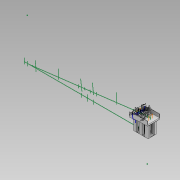
# Autodesk Inventor part: Slope_HighEnd
Saved by Autodesk Inventor 2021 (Build 250183000, 183)
## iProperties
Created: 2021-03-11
Part Number: Slope_HighEnd
Material: 一般
Document SubType Name: Modeling
Designer: kumagai
Density: 1 g/cm^3
Appearance: 既定
Author: kumagai
Autodesk Inventor part; units mm, degrees
ref_plane "YZ Plane" through (0, 0, 0) normal (1, 0, 0) x (0, 1, 0)
ref_plane "XZ Plane" through (0, 0, 0) normal (0, 1, 0) x (-1, 0, 0)
ref_plane "XY Plane" through (0, 0, 0) normal (0, 0, 1) x (1, 0, 0)
derived "SlopeProfile.ipt"
sketch "スケッチ1" plane through (0, 0, 0) normal (0, 0, 1) x (1, 0, 0)
  line L0 (0, 14) -> (0, -14)
  line L1 (-14, 0) -> (14, 0)
  line L2 (-268.75, 0) -> (268.75, 0)
  line L3 (-268.75, 0) -> (268.75, 66)
  line L4 (268.75, 66) -> (268.75, 0)
  line L5 (-31.5879, 61.457) -> (-25.6465, 13.0705)
  line L6 (-134.375, 50.6657) -> (-134.375, 8.5939)
  line L7 (23.2129, 72.7486) -> (28.7067, 28.0077)
  line L8 (-244.2356, 29.1492) -> (-240.1953, -3.7549)
  line L9 (134.375, 89.7324) -> (134.375, 45.3233)
  line L10 (239.1121, 78.5758) -> (241.9591, 55.3901)
  line L11 (-27.6764, 5.7379) -> (-27.6764, -11.9933)
  line L12 (27.6764, 6.5088) -> (27.6764, -13.0212)
  line L13 (-268.75, 0) -> (-295.625, 0)
  line L14 (268.75, 66) -> (295.625, 66)
  line L15 (241.0736, 6.6999) -> (241.0736, -9.2827)
  line L16 (-241.0736, -7.7427) -> (-241.0736, -14.414)
  arc A0 (-280.625, 0) -> (-256.9635, 1.4473) centre (-280.625, 194.1449) ccw
  line L17 (-256.3082, 4.3915) -> (-255.7778, 0.0713)
  line L18 (-280.625, 8.6126) -> (-280.625, -11.6883)
  line L19 (-295.625, 14.7784) -> (-295.625, -11.568)
  line L20 (255.3892, 69.0933) -> (256.9398, 56.465)
  line L21 (280.625, 71.1514) -> (280.625, 58.4982)
  line L22 (295.625, 71.9522) -> (295.625, 60.0478)
  arc A1 (280.625, 66) -> (256.9635, 64.5527) centre (280.625, -128.1449) ccw
  line L23 (-13.2739, 35.3851) -> (-12.039, 25.3288)
  line L24 (-43.1495, 32.5373) -> (-41.4451, 18.6566)
  line L25 (12.2235, 39.1691) -> (13.7539, 26.7059)
  line L26 (41.8424, 44.108) -> (43.6336, 29.5201)
  point P0 (0, 0)
  point P1 (-241.0736, 3.3984)
  point P2 (-27.6764, 29.6016)
  point P3 (27.6764, 36.3984)
  point P4 (241.0736, 62.6016)
  point P5 (134.375, 49.5)
  point P6 (-134.375, 16.5)
ref_plane "作業平面1" through (241.0736, 62.6016, 0) normal (0.9925454, 0.1218753, 0) x (-0.1218753, 0.9925454, 0)
sketch "スケッチ2" plane through (241.0736, 62.6016, 0) normal (0.9925454, 0.1218753, 0) x (-0.1218753, 0.9925454, 0)
  line L0 (16.0942, 0) -> (-7.2657, 0) projected
  line L1 (3.2, 19) -> (-5.2, 19)
  line L2 (-5.2, 19) -> (-5.2, -19)
  line L3 (-5.2, -19) -> (3.2, -19)
  line L4 (3.2, -19) -> (3.2, -17)
  line L5 (3.2, -17) -> (0, -17)
  line L6 (0, -17) -> (0, -9.3)
  line L7 (0, -9.3) -> (3.2, -9.3)
  line L8 (3.2, -9.3) -> (3.2, -6.9)
  line L9 (3.2, -6.9) -> (0, -6.9)
  line L10 (0, -6.9) -> (0, 6.9)
  line L11 (0, 6.9) -> (3.2, 6.9)
  line L12 (3.2, 6.9) -> (3.2, 9.3)
  line L13 (3.2, 9.3) -> (0, 9.3)
  line L14 (0, 9.3) -> (0, 17)
  line L15 (0, 17) -> (3.2, 17)
  line L16 (3.2, 17) -> (3.2, 19)
  line L17 (-5.2, 27.5) -> (-5.2, -27.5)
  line L18 (-5.2, -27.5) -> (9, -27.5)
  line L19 (9, -27.5) -> (9, -29.5)
  line L20 (9, -29.5) -> (-11, -29.5)
  line L21 (-11, -29.5) -> (-11, 29.5)
  line L22 (-11, 29.5) -> (9, 29.5)
  line L23 (9, 29.5) -> (9, 27.5)
  line L24 (9, 27.5) -> (-5.2, 27.5)
  line L25 (-11, -29.5) -> (-20.0203, -18.75)
  line L26 (-20.0203, -18.75) -> (-31, -18.75)
  line L27 (-31, -18.75) -> (-31, -10.75)
  line L28 (-31, -10.75) -> (-20.0203, -10.75)
  line L29 (-20.0203, -10.75) -> (-11, 0)
  line L30 (-11, 0) -> (-20.0203, 10.75)
  line L31 (-20.0203, 10.75) -> (-31, 10.75)
  line L32 (-31, 10.75) -> (-31, 18.75)
  line L33 (-31, 18.75) -> (-20.0203, 18.75)
  line L34 (-20.0203, 18.75) -> (-11, 29.5)
  point P0 (-32.754, 0)
  point P1 (0, 0)
  point P2 (-5.2, 19)
  point P3 (-5.2, -19)
  dimension "d14" = 27.6764
  dimension "d25" = 38
  dimension "d26" = 8.4
  dimension "d27" = 3.2
  dimension "d28" = 18.6
  dimension "d29" = 2.4
  dimension "d30" = 2
  dimension "d31" = 59
  dimension "d32" = 2
  dimension "d33" = 20
  dimension "d34" = 5.8
  dimension "d36" = 5.8
  dimension "d53" = 40
  dimension "d54" = 40
  dimension "d55" = 8
  dimension "d56" = 20
  constraints: 68 end point, 21 perpendicular, 6 point on line, 3 collinear, 3 horizontal, 3 vertical, 2 midpoint, 1 parallel, 1 vertical alignment, 11 other
  measures "d25" distance between parallel lines of L3 L1
  measures "d26" distance between parallel lines of L2 L4
  measures "d27" distance between parallel lines of L6 L4
  measures "d28" distance between parallel lines of L7 L13
  measures "d29" distance between parallel lines of L13 L11
  measures "d30" distance between parallel lines of L1 L15
  measures "d31" distance between parallel lines of L22 L20
  measures "d32" distance between parallel lines of L22 L24
  measures "d33" distance between parallel lines of L21 L19
  measures "d34" distance between parallel lines of L4 L19
  measures "d36" distance between parallel lines of L21 L17
  measures "d53" angle of L21 L25
  measures "d54" angle of L21 L29
  measures "d55" distance between parallel lines of L28 L26
  measures "d56" distance between parallel lines of L27 L21
sketch "スケッチ3" plane through (0, 0, 0) normal (0, 0, 1) x (1, 0, 0)
  arc A0 (280.625, 66) -> (256.9635, 64.5527) centre (280.625, -128.1449) ccw projected
  line L0 (-268.75, 0) -> (268.75, 66) projected
  line L1 (256.9635, 64.5527) -> (226.1855, 60.7735)
  line L2 (239.1121, 78.5758) -> (241.9591, 55.3901) projected
  line L3 (280.625, 66) -> (310.625, 66)
  line L4 (295.625, 71.9522) -> (295.625, 60.0478) projected
  point P0 (0, 0)
  dimension "d14" = 27.6764
  dimension "d37" = 15
  dimension "d39" = 15
  constraints: 4 end point, 1 horizontal, 1 point on line
  measures "d37" distance from line of L1.end L2
  measures "d39" distance from line of L3.end L4
sweep "スイープ1" add profiles "スケッチ2" path "スケッチ3" path curves L1 A0 L3
extrude "押し出し1" cut sketch "スケッチ2" along normal blind 15 and the other way blind 15 contours L10 L9 L8 L7 L6 L5 L4 L3 L2 L0 | L0 L2 L1 L16 L15 L14 L13 L12 L11 L10
ref_plane "作業平面2" through (295.625, 66, 0) normal (1, 0, 0) x (0, 1, 0)
sketch "スケッチ4" plane through (295.625, 66, 0) normal (1, 0, 0) x (0, 1, 0)
  line L0 (3.2, 19.5) -> (-5.2, 19.5)
  line L1 (-5.2, 19.5) -> (-5.2, -19.5)
  line L2 (-5.2, -19.5) -> (3.2, -19.5)
  line L3 (3.2, -19.5) -> (3.2, 19.5)
  line L4 (5.9522, 0) -> (-5.9522, 0) projected
  point P0 (-66, 0)
  point P1 (0, 0)
  dimension "d14" = 27.6764
  dimension "d46" = 39
  dimension "d47" = 3.2
  dimension "d48" = 8.4
  constraints: 8 end point, 2 parallel, 1 horizontal, 1 perpendicular, 1 other
  measures "d46" distance between parallel lines of L2 L0
  measures "d47" distance from line of point (0, 0) L3
  measures "d48" distance between parallel lines of L1 L3
extrude "押し出し2" cut sketch "スケッチ4" along normal blind 15 and the other way blind 15
sketch "スケッチ5" plane through (295.625, 66, 0) normal (1, 0, 0) x (0, 1, 0)
  line L0 (-66, 41.3) -> (-66, -41.3) projected
  line L1 (-20.0203, 18.75) -> (-71.2, 18.75)
  line L2 (-71.2, 18.75) -> (-71.2, 10.75)
  line L3 (-69.2, 10.75) -> (-20.0203, 10.75)
  line L4 (-20.0203, 10.75) -> (-20.0203, 18.75)
  line L5 (-21.3183, -18.75) -> (-20.0203, -18.75) projected
  line L6 (-20.0203, -18.75) -> (-71.2, -18.75)
  line L7 (-71.2, -18.75) -> (-71.2, -10.75)
  line L8 (-69.2, -10.75) -> (-20.0203, -10.75)
  line L9 (-20.0203, -10.75) -> (-20.0203, -18.75)
  line L10 (-258.6029, 0) -> (192.6029, 0) projected
  line L11 (-71.2, -10.75) -> (-71.2, 10.75)
  line L12 (-69.2, -10.75) -> (-69.2, 10.75)
  point P0 (-66, 0)
  dimension "d57" = 5.2
  dimension "d76" = 2
  constraints: 20 end point, 5 parallel, 2 horizontal, 2 perpendicular, 2 point on line, 1 vertical, 2 other
  measures "d57" distance between parallel lines of L0 L2
  measures "d76" distance between parallel lines of L11 L12
extrude "押し出し3" add sketch "スケッチ5" along normal blind 15 and the other way blind 70 contours L1 L4 L3 L0 | L0 L3 L12 L10 L11 L2 L1 | L8 L9 L5 L6 L0 | L0 L6 L7 L11 L10 L12 L8
sketch "スケッチ6" plane through (0, 0, 0) normal (0, 0, 1) x (1, 0, 0)
  line L0 (228.6254, 40.9024) -> (259.4035, 44.6817) projected
  arc A0 (280.625, 45.9797) -> (259.4035, 44.6817) centre (280.625, -128.1449) ccw projected
  line L1 (280.625, 45.9797) -> (310.625, 45.9797) projected
  line L2 (227.5261, 49.8555) -> (234.4396, 41.6163)
  line L3 (234.4396, 41.6163) -> (234.4396, -5.2)
  line L4 (310.625, 55) -> (303.0561, 45.9797)
  line L5 (303.0561, 45.9797) -> (303.0561, -5.2)
  line L6 (227.5261, 49.8555) -> (222.5261, 49.8555)
  line L7 (222.5261, 49.8555) -> (222.5261, -5.2)
  line L8 (222.5261, -5.2) -> (234.4472, -5.2)
  line L9 (310.625, 55) -> (310.625, 45.9797) projected
  line L10 (310.625, 55) -> (315.625, 55)
  line L11 (315.625, 55) -> (315.625, -5.2)
  line L12 (315.625, -5.2) -> (303.0561, -5.2)
  line L13 (228.6254, 40.9024) -> (259.4035, 44.6817) projected
  line L14 (280.625, 45.9797) -> (310.625, 45.9797) projected
  line L15 (249.4396, 43.4582) -> (249.4396, -3.2)
  line L16 (249.4396, -3.2) -> (261.25, -3.2)
  line L17 (261.25, -3.2) -> (261.25, 44.8984)
  line L18 (276.25, 45.9247) -> (276.25, -3.2)
  line L19 (276.25, -3.2) -> (288.0604, -3.2)
  line L20 (288.0604, -3.2) -> (288.0604, 45.9797)
  line L21 (268.75, 66) -> (268.75, 0) projected
  line L22 (227.5261, 49.8555) -> (258.3042, 53.6347) projected
  line L23 (280.625, 55) -> (310.625, 55) projected
  line L24 (255.3448, 53.2713) -> (249.4396, 43.4582)
  line L25 (255.3448, 53.2713) -> (261.25, 44.8984)
  line L26 (282.1552, 55) -> (276.25, 45.9247)
  line L27 (282.1552, 55) -> (288.0604, 45.9797)
  line L28 (225.625, -5.2) -> (310.625, -5.2) projected
  point P0 (0, 0)
  point P1 (234.4396, -5.2)
  dimension "d64" = 5
  dimension "d65" = 5
  dimension "d66" = 15
  dimension "d67" = 15
  dimension "d68" = 5.9052
  dimension "d69" = 5.9052
  dimension "d70" = 5.9052
  dimension "d71" = 5.9052
  dimension "d77" = 2
  dimension "d78" = 2
  constraints: 40 end point, 6 point on line, 4 horizontal, 3 perpendicular, 2 collinear, 2 point on circle, 1 vertical, 2 other
  measures "d64" distance of L2.start L6.end
  measures "d65" distance of L4.start L10.end
  measures "d66" distance between parallel lines of L18 L17
  measures "d67" distance between parallel lines of L3 L15
  measures "d68" distance from line of L24.start L15
  measures "d69" distance from line of L24.start L17
  measures "d70" distance from line of L26.start L18
  measures "d71" distance from line of L26.start L20
  measures "d77" distance between parallel lines of L28 L16
  measures "d78" distance between parallel lines of L28 L19
extrude "押し出し4" cut sketch "スケッチ6" against normal through all both and the other way through all contours L3 L8 L7 L6 L2 | L24 L25 A0 L0 | L0 A0 L17 L16 L15 | L5 L1 L9 L10 L11 L12 | L4 L9 L1 | L26 L27 L1 A0 | A0 L1 L20 L19 L18
equation "\"d25\" = RailWidth"
equation "\"d26\" = RailHeight"
equation "\"d27\" = RailDepth"
equation "\"d28\" = InsideWidth"
equation "\"d29\" = InnerWall"
equation "\"d30\" = OuterWall"
equation "\"d34\" = d36"
equation "\"d42\" = ConnectorLength"
equation "\"d47\" = RailDepth"
equation "\"d48\" = RailHeight"
equation "\"d50\" = ConnectorLength"
equation "\"d57\" = RailHeight - RailDepth"
equation "\"d68\" = d69"
equation "\"d70\" = d71"
equation "\"RailWidth\" = 38"
equation "\"RailHeight\" = 8.4"
equation "\"RailDepth\" = 3.2"
equation "\"InsideWidth\" = 18.6"
equation "\"InnerWall\" = 2.4"
equation "\"OuterWall\" = 2"
equation "\"ConnectorLength\" = 15"
